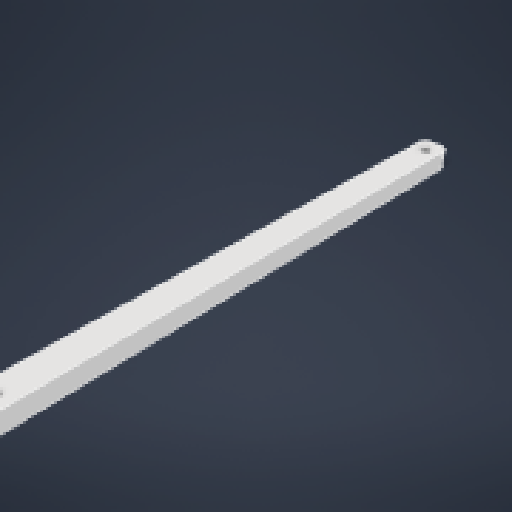
# Autodesk Inventor part: Steering_Servo_Linkage
Saved by Autodesk Inventor 2025 (Build 290162000, 162)
## iProperties
Created: 2024-05-24
Part Number: Steering_Servo_Linkage
Material: Generic
Document SubType Name: Modeling
Designer: Garfieldcmix
Density: 1 g/cm^3
Appearance: Default
Author: Garfieldcmix
Autodesk Inventor part; units mm, degrees
ref_plane "YZ Plane" through (0, 0, 0) normal (1, 0, 0) x (0, 1, 0)
ref_plane "XZ Plane" through (0, 0, 0) normal (0, 1, 0) x (-1, 0, 0)
ref_plane "XY Plane" through (0, 0, 0) normal (0, 0, 1) x (1, 0, 0)
sketch "Sketch1" plane through (0, 0, 0) normal (0, 1, 0) x (-1, 0, 0)
  line L0 (0, 0) -> (3, 0)
  line L1 (3, 0) -> (3, -52)
  line L2 (3, -52) -> (0, -52)
  line L3 (0, -52) -> (0, 0)
  circle A0 centre (1.5, -2) radius 0.6
  circle A1 centre (1.5, -50) radius 0.6
  point P0 (1.5, 0)
  dimension "d0" = 3
  dimension "d1" = 52
  dimension "d2" = 1.2
  dimension "d3" = 1.2
  dimension "d4" = 48
  dimension "d5" = 1.5
  dimension "d6" = 1.5
  dimension "d7" = 2
  constraints: 8 end point, 2 centre point, 2 parallel, 1 horizontal, 1 midpoint, 1 perpendicular
  measures "d0" distance of L1.end L2.end
  measures "d1" distance of L0.end L1.end
  measures "d2" diameter of A0
  measures "d3" diameter of A1
  measures "d4" distance of A1.centre A0.centre
  measures "d5" distance from line of L1 A0.centre
  measures "d6" distance from line of L1 A1.centre
  measures "d7" distance of point (1.5, 0) A0.centre
extrude "Extrusion1" add sketch "Sketch1" along normal blind 2
fillet "Fillet1" radius 1 4 edges at (0, 1, 0) (-3, 1, 0) (0, 1, -52) (-3, 1, -52)
equation "\"d5\" = 0.5 * d0"
equation "\"d6\" = d5"
body "Solid1"
